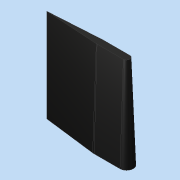
# Autodesk Inventor part: GenericControlSurface
Saved by Autodesk Inventor 2017 (Build 210142000, 142)
## iProperties
Created: 2016-10-11
Part Number: GenericControlSurface
Material: Generic
Document SubType Name: Modeling
Designer: techn
Density: 1 g/cm^3
Appearance: Glossy - Black
Author: techn
Autodesk Inventor part; units mm, degrees
ref_plane "YZ Plane" through (0, 0, 0) normal (1, 0, 0) x (0, 1, 0)
ref_plane "XY Plane" through (0, 0, 0) normal (0, 0, 1) x (1, 0, 0)
sketch "Sketch2" plane through (0, 0, 0) normal (0, 1, 0) x (-1, 0, 0)
  circle A0 centre (0, 0) radius 3.175
  line L0 (0, 0) -> (38.1, 0)
  line L1 (0, 3.175) -> (12.3047, 3.175)
  line L2 (0, -3.175) -> (12.3047, -3.175)
  line L3 (13.0923, -3.126) -> (38.1, 0)
  line L4 (38.1, 0) -> (13.0923, 3.126)
  arc A1 (13.0923, 3.126) -> (12.3047, 3.175) centre (12.3047, -3.175) ccw
  arc A2 (12.3047, -3.175) -> (13.0923, -3.126) centre (12.3047, 3.175) ccw
  circle A3 centre (0, 0) radius 1.5875
  point P0 (12.7, 3.175)
  dimension "d5" = 6.35
  dimension "d6" = 38.1
  dimension "d7" = 12.7
  dimension "d8" = 6.35
  dimension "d9" = 6.35
  dimension "d12" = 3.175
  constraints: 10 end point, 6 point on circle, 5 tangent, 4 centre point, 3 horizontal, 2 coincident, 2 point on line
  measures "d5" diameter of A0
  measures "d6" distance of L0.start L0.end
  measures "d7" distance of L1.start point (12.7, 3.175)
  measures "d8" radius of A1
  measures "d9" radius of A2
  measures "d12" diameter of A3
ref_plane "Work Plane1" through (0, 44.45, 0) normal (0, 1, 0) x (-1, 0, 0)
sketch "Sketch3" plane through (0, 44.45, 0) normal (0, 1, 0) x (-1, 0, 0)
  circle A0 centre (0, 0) radius 1.5875
  line L0 (0, 1.5875) -> (12.5018, 1.5875)
  line L1 (0, -1.5875) -> (12.5018, -1.5875)
  line L2 (12.8979, -1.5751) -> (38.1, 0)
  line L3 (38.1, 0) -> (12.8979, 1.5751)
  arc A1 (12.8979, 1.5751) -> (12.5018, 1.5875) centre (12.5018, -4.7625) ccw
  arc A2 (12.5018, -1.5875) -> (12.8979, -1.5751) centre (12.5018, 4.7625) ccw
  point P0 (12.7, 1.5875)
  dimension "d14" = 3.175
  dimension "d15" = 12.7
  dimension "d16" = 6.35
  dimension "d17" = 6.35
  constraints: 8 end point, 6 point on circle, 6 tangent, 3 centre point, 2 horizontal, 2 point on line, 1 coincident
  measures "d14" diameter of A0
  measures "d15" distance of L0.start point (12.7, 1.587)
  measures "d16" radius of A1
  measures "d17" radius of A2
loft "Loft1" add profiles "Sketch2", "Sketch3" contours A0 | L0 L3 A2 L2 A0 | A0 L1 A1 L4 L0 | A3 / all
sketch "Sketch4" plane through (0, 0, 0) normal (0, 0, 1) x (1, 0, 0)
  line L0 (-12.3047, 0) -> (0, 0) projected
  line L1 (0, 0) -> (0, 12.7)
  line L2 (0, 0) -> (0, 44.45) projected
  line L3 (0, 12.7) -> (-7.9375, 12.7)
  line L4 (-7.9375, 12.7) -> (-7.9375, 20.6375)
  arc A0 (0, 12.7) -> (-7.9375, 20.6375) centre (-7.9375, 12.7) ccw
  line L5 (-7.9375, 20.6375) -> (-14.2875, 20.6375)
  dimension "d22" = 12.7
  dimension "d23" = 7.9375
  dimension "d24" = 7.9375
  dimension "d25" = 6.35
  constraints: 8 end point, 2 horizontal, 2 point on circle, 1 centre point, 1 point on line, 1 tangent, 1 vertical
  measures "d22" distance of L0.end L1.end
  measures "d23" distance of L1.end L3.end
  measures "d24" distance of L3.end L4.end
  measures "d25" distance of L4.end L5.end
sketch "Sketch5" plane through (-12.3047, 0, -3.175) normal (0, -1, 0) x (1, 0, 0)
  circle A0 centre (12.3047, 3.175) radius 1.5875
  dimension "d26" = 3.175
  constraints: 1 centre point, 1 coincident
  measures "d26" diameter of A0
sweep "Sweep1" cut profiles "Sketch5" path "Sketch4" path curves L1 A0 L5
body "Solid3"
